Autodesk Fusion 360 part; units mm, degrees
(part 9 of 12)
  arc A1435 (77.1012, -97.0282) -> (78.6012, -97.0282) centre (77.8512, -97.0282) ccw
  arc A1436 (78.6012, -97.0282) -> (77.1012, -97.0282) centre (77.8512, -97.0282) ccw
  arc A1437 (77.1012, -97.0282) -> (78.6012, -97.0282) centre (77.8512, -97.0282) ccw
  arc A1438 (45.5811, -89.4082) -> (44.0811, -89.4082) centre (44.8311, -89.4082) ccw
  arc A1439 (44.0811, -89.4082) -> (45.5811, -89.4082) centre (44.8311, -89.4082) ccw
  arc A1440 (45.5811, -89.4082) -> (44.0811, -89.4082) centre (44.8311, -89.4082) ccw
  arc A1441 (44.0811, -89.4082) -> (45.5811, -89.4082) centre (44.8311, -89.4082) ccw
  arc A1442 (44.0811, -89.4082) -> (45.5811, -89.4082) centre (44.8311, -89.4082) ccw
  arc A1443 (45.5811, -89.4082) -> (44.0811, -89.4082) centre (44.8311, -89.4082) ccw
  arc A1444 (46.6211, -89.4082) -> (48.1211, -89.4082) centre (47.3711, -89.4082) ccw
  arc A1445 (48.1211, -89.4082) -> (46.6211, -89.4082) centre (47.3711, -89.4082) ccw
  arc A1446 (48.1211, -89.4082) -> (46.6211, -89.4082) centre (47.3711, -89.4082) ccw
  arc A1447 (46.6211, -89.4082) -> (48.1211, -89.4082) centre (47.3711, -89.4082) ccw
  arc A1448 (46.6211, -89.4082) -> (48.1211, -89.4082) centre (47.3711, -89.4082) ccw
  arc A1449 (48.1211, -89.4082) -> (46.6211, -89.4082) centre (47.3711, -89.4082) ccw
  arc A1450 (49.1611, -89.4082) -> (50.6611, -89.4082) centre (49.9111, -89.4082) ccw
  arc A1451 (50.6611, -89.4082) -> (49.1611, -89.4082) centre (49.9111, -89.4082) ccw
  arc A1452 (50.6611, -89.4082) -> (49.1611, -89.4082) centre (49.9111, -89.4082) ccw
  arc A1453 (49.1611, -89.4082) -> (50.6611, -89.4082) centre (49.9111, -89.4082) ccw
  arc A1454 (49.1611, -89.4082) -> (50.6611, -89.4082) centre (49.9111, -89.4082) ccw
  arc A1455 (50.6611, -89.4082) -> (49.1611, -89.4082) centre (49.9111, -89.4082) ccw
  arc A1456 (53.2011, -89.4082) -> (51.7011, -89.4082) centre (52.4511, -89.4082) ccw
  arc A1457 (51.7011, -89.4082) -> (53.2011, -89.4082) centre (52.4511, -89.4082) ccw
  arc A1458 (51.7011, -89.4082) -> (53.2011, -89.4082) centre (52.4511, -89.4082) ccw
  arc A1459 (53.2011, -89.4082) -> (51.7011, -89.4082) centre (52.4511, -89.4082) ccw
  arc A1460 (53.2011, -89.4082) -> (51.7011, -89.4082) centre (52.4511, -89.4082) ccw
  arc A1461 (51.7011, -89.4082) -> (53.2011, -89.4082) centre (52.4511, -89.4082) ccw
  arc A1462 (55.7411, -89.4082) -> (54.2411, -89.4082) centre (54.9911, -89.4082) ccw
  arc A1463 (54.2411, -89.4082) -> (55.7411, -89.4082) centre (54.9911, -89.4082) ccw
  arc A1464 (55.7411, -89.4082) -> (54.2411, -89.4082) centre (54.9911, -89.4082) ccw
  arc A1465 (54.2411, -89.4082) -> (55.7411, -89.4082) centre (54.9911, -89.4082) ccw
  arc A1466 (55.7411, -89.4082) -> (54.2411, -89.4082) centre (54.9911, -89.4082) ccw
  arc A1467 (54.2411, -89.4082) -> (55.7411, -89.4082) centre (54.9911, -89.4082) ccw
  arc A1468 (56.7811, -89.4082) -> (58.2811, -89.4082) centre (57.5311, -89.4082) ccw
  arc A1469 (58.2811, -89.4082) -> (56.7811, -89.4082) centre (57.5311, -89.4082) ccw
  arc A1470 (56.7811, -89.4082) -> (58.2811, -89.4082) centre (57.5311, -89.4082) ccw
  arc A1471 (58.2811, -89.4082) -> (56.7811, -89.4082) centre (57.5311, -89.4082) ccw
  arc A1472 (58.2811, -89.4082) -> (56.7811, -89.4082) centre (57.5311, -89.4082) ccw
  arc A1473 (56.7811, -89.4082) -> (58.2811, -89.4082) centre (57.5311, -89.4082) ccw
  arc A1474 (60.8211, -89.4082) -> (59.3211, -89.4082) centre (60.0711, -89.4082) ccw
  arc A1475 (59.3211, -89.4082) -> (60.8211, -89.4082) centre (60.0711, -89.4082) ccw
  arc A1476 (60.8211, -89.4082) -> (59.3211, -89.4082) centre (60.0711, -89.4082) ccw
  arc A1477 (59.3211, -89.4082) -> (60.8211, -89.4082) centre (60.0711, -89.4082) ccw
  arc A1478 (60.8211, -89.4082) -> (59.3211, -89.4082) centre (60.0711, -89.4082) ccw
  arc A1479 (59.3211, -89.4082) -> (60.8211, -89.4082) centre (60.0711, -89.4082) ccw
  arc A1480 (61.8611, -89.4082) -> (63.3611, -89.4082) centre (62.6111, -89.4082) ccw
  arc A1481 (63.3611, -89.4082) -> (61.8611, -89.4082) centre (62.6111, -89.4082) ccw
  arc A1482 (63.3611, -89.4082) -> (61.8611, -89.4082) centre (62.6111, -89.4082) ccw
  arc A1483 (61.8611, -89.4082) -> (63.3611, -89.4082) centre (62.6111, -89.4082) ccw
  arc A1484 (63.3611, -89.4082) -> (61.8611, -89.4082) centre (62.6111, -89.4082) ccw
  arc A1485 (61.8611, -89.4082) -> (63.3611, -89.4082) centre (62.6111, -89.4082) ccw
  arc A1486 (65.9011, -89.4082) -> (64.4011, -89.4082) centre (65.1511, -89.4082) ccw
  arc A1487 (64.4011, -89.4082) -> (65.9011, -89.4082) centre (65.1511, -89.4082) ccw
  arc A1488 (64.4011, -89.4082) -> (65.9011, -89.4082) centre (65.1511, -89.4082) ccw
  arc A1489 (65.9011, -89.4082) -> (64.4011, -89.4082) centre (65.1511, -89.4082) ccw
  arc A1490 (64.4011, -89.4082) -> (65.9011, -89.4082) centre (65.1511, -89.4082) ccw
  arc A1491 (65.9011, -89.4082) -> (64.4011, -89.4082) centre (65.1511, -89.4082) ccw
  arc A1492 (68.4411, -89.4082) -> (66.9411, -89.4082) centre (67.6911, -89.4082) ccw
  arc A1493 (66.9411, -89.4082) -> (68.4411, -89.4082) centre (67.6911, -89.4082) ccw
  arc A1494 (68.4411, -89.4082) -> (66.9411, -89.4082) centre (67.6911, -89.4082) ccw
  arc A1495 (66.9411, -89.4082) -> (68.4411, -89.4082) centre (67.6911, -89.4082) ccw
  arc A1496 (66.9411, -89.4082) -> (68.4411, -89.4082) centre (67.6911, -89.4082) ccw
  arc A1497 (68.4411, -89.4082) -> (66.9411, -89.4082) centre (67.6911, -89.4082) ccw
  arc A1498 (69.4811, -89.4082) -> (70.9811, -89.4082) centre (70.2311, -89.4082) ccw
  arc A1499 (70.9811, -89.4082) -> (69.4811, -89.4082) centre (70.2311, -89.4082) ccw
  arc A1500 (69.4811, -89.4082) -> (70.9811, -89.4082) centre (70.2311, -89.4082) ccw
  arc A1501 (70.9811, -89.4082) -> (69.4811, -89.4082) centre (70.2311, -89.4082) ccw
  arc A1502 (69.4811, -89.4082) -> (70.9811, -89.4082) centre (70.2311, -89.4082) ccw
  arc A1503 (70.9811, -89.4082) -> (69.4811, -89.4082) centre (70.2311, -89.4082) ccw
  arc A1504 (72.0211, -89.4082) -> (73.5211, -89.4082) centre (72.7711, -89.4082) ccw
  arc A1505 (73.5211, -89.4082) -> (72.0211, -89.4082) centre (72.7711, -89.4082) ccw
  arc A1506 (73.5211, -89.4082) -> (72.0211, -89.4082) centre (72.7711, -89.4082) ccw
  arc A1507 (72.0211, -89.4082) -> (73.5211, -89.4082) centre (72.7711, -89.4082) ccw
  arc A1508 (72.0211, -89.4082) -> (73.5211, -89.4082) centre (72.7711, -89.4082) ccw
  arc A1509 (73.5211, -89.4082) -> (72.0211, -89.4082) centre (72.7711, -89.4082) ccw
  arc A1510 (76.0612, -89.4082) -> (74.5612, -89.4082) centre (75.3112, -89.4082) ccw
  arc A1511 (74.5612, -89.4082) -> (76.0612, -89.4082) centre (75.3112, -89.4082) ccw
  arc A1512 (74.5612, -89.4082) -> (76.0612, -89.4082) centre (75.3112, -89.4082) ccw
  arc A1513 (76.0612, -89.4082) -> (74.5612, -89.4082) centre (75.3112, -89.4082) ccw
  arc A1514 (76.0612, -89.4082) -> (74.5612, -89.4082) centre (75.3112, -89.4082) ccw
  arc A1515 (74.5612, -89.4082) -> (76.0612, -89.4082) centre (75.3112, -89.4082) ccw
  line L256 (77.1012, -90.1582) -> (77.1012, -88.6582)
  line L257 (77.1012, -88.6582) -> (78.6012, -88.6582)
  line L258 (78.6012, -88.6582) -> (78.6012, -90.1582)
  line L259 (78.6012, -90.1582) -> (77.1012, -90.1582)
  line L260 (77.1012, -90.1582) -> (77.1012, -88.6582)
  line L261 (78.6012, -90.1582) -> (77.1012, -90.1582)
  line L262 (77.1012, -88.6582) -> (78.6012, -88.6582)
  line L263 (78.6012, -88.6582) -> (78.6012, -90.1582)
  line L264 (77.1012, -88.6582) -> (78.6012, -88.6582)
  line L265 (77.1012, -90.1582) -> (77.1012, -88.6582)
  line L266 (78.6012, -90.1582) -> (77.1012, -90.1582)
  line L267 (78.6012, -88.6582) -> (78.6012, -90.1582)
  arc A1516 (-155.9813, -117.1772) -> (-153.4413, -117.1772) centre (-154.7113, -117.1772) ccw
  arc A1517 (-153.4413, -117.1772) -> (-155.9813, -117.1772) centre (-154.7113, -117.1772) ccw
  arc A1518 (-153.4413, -117.1772) -> (-155.9813, -117.1772) centre (-154.7113, -117.1772) ccw
  arc A1519 (-155.9813, -117.1772) -> (-153.4413, -117.1772) centre (-154.7113, -117.1772) ccw
  arc A1520 (-153.4413, -117.1772) -> (-155.9813, -117.1772) centre (-154.7113, -117.1772) ccw
  arc A1521 (-155.9813, -117.1772) -> (-153.4413, -117.1772) centre (-154.7113, -117.1772) ccw
  arc A1522 (-159.7913, -119.7172) -> (-162.3313, -119.7172) centre (-161.0613, -119.7172) ccw
  arc A1523 (-162.3313, -119.7172) -> (-159.7913, -119.7172) centre (-161.0613, -119.7172) ccw
  arc A1524 (-159.7913, -119.7172) -> (-162.3313, -119.7172) centre (-161.0613, -119.7172) ccw
  arc A1525 (-162.3313, -119.7172) -> (-159.7913, -119.7172) centre (-161.0613, -119.7172) ccw
  arc A1526 (-159.7913, -119.7172) -> (-162.3313, -119.7172) centre (-161.0613, -119.7172) ccw
  arc A1527 (-162.3313, -119.7172) -> (-159.7913, -119.7172) centre (-161.0613, -119.7172) ccw
  arc A1528 (-110.7819, -117.1772) -> (-113.3219, -117.1772) centre (-112.0519, -117.1772) ccw
  arc A1529 (-113.3219, -117.1772) -> (-110.7819, -117.1772) centre (-112.0519, -117.1772) ccw
  arc A1530 (-113.3219, -117.1772) -> (-110.7819, -117.1772) centre (-112.0519, -117.1772) ccw
  arc A1531 (-110.7819, -117.1772) -> (-113.3219, -117.1772) centre (-112.0519, -117.1772) ccw
  arc A1532 (-113.3219, -117.1772) -> (-110.7819, -117.1772) centre (-112.0519, -117.1772) ccw
  arc A1533 (-110.7819, -117.1772) -> (-113.3219, -117.1772) centre (-112.0519, -117.1772) ccw
  arc A1534 (-117.132, -119.7172) -> (-119.672, -119.7172) centre (-118.402, -119.7172) ccw
  arc A1535 (-119.672, -119.7172) -> (-117.132, -119.7172) centre (-118.402, -119.7172) ccw
  arc A1536 (-117.132, -119.7172) -> (-119.672, -119.7172) centre (-118.402, -119.7172) ccw
  arc A1537 (-119.672, -119.7172) -> (-117.132, -119.7172) centre (-118.402, -119.7172) ccw
  arc A1538 (-117.132, -119.7172) -> (-119.672, -119.7172) centre (-118.402, -119.7172) ccw
  arc A1539 (-119.672, -119.7172) -> (-117.132, -119.7172) centre (-118.402, -119.7172) ccw
  arc A1540 (-80.7819, -117.1772) -> (-83.3219, -117.1772) centre (-82.0519, -117.1772) ccw
  arc A1541 (-83.3219, -117.1772) -> (-80.7819, -117.1772) centre (-82.0519, -117.1772) ccw
  arc A1542 (-83.3219, -117.1772) -> (-80.7819, -117.1772) centre (-82.0519, -117.1772) ccw
  arc A1543 (-80.7819, -117.1772) -> (-83.3219, -117.1772) centre (-82.0519, -117.1772) ccw
  arc A1544 (-83.3219, -117.1772) -> (-80.7819, -117.1772) centre (-82.0519, -117.1772) ccw
  arc A1545 (-80.7819, -117.1772) -> (-83.3219, -117.1772) centre (-82.0519, -117.1772) ccw
  arc A1546 (-89.672, -119.7172) -> (-87.132, -119.7172) centre (-88.402, -119.7172) ccw
  arc A1547 (-87.132, -119.7172) -> (-89.672, -119.7172) centre (-88.402, -119.7172) ccw
  arc A1548 (-87.132, -119.7172) -> (-89.672, -119.7172) centre (-88.402, -119.7172) ccw
  arc A1549 (-89.672, -119.7172) -> (-87.132, -119.7172) centre (-88.402, -119.7172) ccw
  arc A1550 (-87.132, -119.7172) -> (-89.672, -119.7172) centre (-88.402, -119.7172) ccw
  arc A1551 (-89.672, -119.7172) -> (-87.132, -119.7172) centre (-88.402, -119.7172) ccw
  arc A1552 (-53.3219, -117.1772) -> (-50.7819, -117.1772) centre (-52.0519, -117.1772) ccw
  arc A1553 (-50.7819, -117.1772) -> (-53.3219, -117.1772) centre (-52.0519, -117.1772) ccw
  arc A1554 (-50.7819, -117.1772) -> (-53.3219, -117.1772) centre (-52.0519, -117.1772) ccw
  arc A1555 (-53.3219, -117.1772) -> (-50.7819, -117.1772) centre (-52.0519, -117.1772) ccw
  arc A1556 (-50.7819, -117.1772) -> (-53.3219, -117.1772) centre (-52.0519, -117.1772) ccw
  arc A1557 (-53.3219, -117.1772) -> (-50.7819, -117.1772) centre (-52.0519, -117.1772) ccw
  arc A1558 (-57.132, -119.7172) -> (-59.672, -119.7172) centre (-58.402, -119.7172) ccw
  arc A1559 (-59.672, -119.7172) -> (-57.132, -119.7172) centre (-58.402, -119.7172) ccw
  arc A1560 (-57.132, -119.7172) -> (-59.672, -119.7172) centre (-58.402, -119.7172) ccw
  arc A1561 (-59.672, -119.7172) -> (-57.132, -119.7172) centre (-58.402, -119.7172) ccw
  arc A1562 (-57.132, -119.7172) -> (-59.672, -119.7172) centre (-58.402, -119.7172) ccw
  arc A1563 (-59.672, -119.7172) -> (-57.132, -119.7172) centre (-58.402, -119.7172) ccw
  arc A1564 (-23.3219, -117.1772) -> (-20.7819, -117.1772) centre (-22.0519, -117.1772) ccw
  arc A1565 (-20.7819, -117.1772) -> (-23.3219, -117.1772) centre (-22.0519, -117.1772) ccw
  arc A1566 (-20.7819, -117.1772) -> (-23.3219, -117.1772) centre (-22.0519, -117.1772) ccw
  arc A1567 (-23.3219, -117.1772) -> (-20.7819, -117.1772) centre (-22.0519, -117.1772) ccw
  arc A1568 (-20.7819, -117.1772) -> (-23.3219, -117.1772) centre (-22.0519, -117.1772) ccw
  arc A1569 (-23.3219, -117.1772) -> (-20.7819, -117.1772) centre (-22.0519, -117.1772) ccw
  arc A1570 (-27.132, -119.7172) -> (-29.672, -119.7172) centre (-28.402, -119.7172) ccw
  arc A1571 (-29.672, -119.7172) -> (-27.132, -119.7172) centre (-28.402, -119.7172) ccw
  arc A1572 (-27.132, -119.7172) -> (-29.672, -119.7172) centre (-28.402, -119.7172) ccw
  arc A1573 (-29.672, -119.7172) -> (-27.132, -119.7172) centre (-28.402, -119.7172) ccw
  arc A1574 (-27.132, -119.7172) -> (-29.672, -119.7172) centre (-28.402, -119.7172) ccw
  arc A1575 (-29.672, -119.7172) -> (-27.132, -119.7172) centre (-28.402, -119.7172) ccw
  arc A1576 (6.6781, -117.1772) -> (9.2181, -117.1772) centre (7.9481, -117.1772) ccw
  arc A1577 (9.2181, -117.1772) -> (6.6781, -117.1772) centre (7.9481, -117.1772) ccw
  arc A1578 (6.6781, -117.1772) -> (9.2181, -117.1772) centre (7.9481, -117.1772) ccw
  arc A1579 (9.2181, -117.1772) -> (6.6781, -117.1772) centre (7.9481, -117.1772) ccw
  arc A1580 (6.6781, -117.1772) -> (9.2181, -117.1772) centre (7.9481, -117.1772) ccw
  arc A1581 (9.2181, -117.1772) -> (6.6781, -117.1772) centre (7.9481, -117.1772) ccw
  arc A1582 (2.868, -119.7172) -> (0.328, -119.7172) centre (1.598, -119.7172) ccw
  arc A1583 (0.328, -119.7172) -> (2.868, -119.7172) centre (1.598, -119.7172) ccw
  arc A1584 (2.868, -119.7172) -> (0.328, -119.7172) centre (1.598, -119.7172) ccw
  arc A1585 (0.328, -119.7172) -> (2.868, -119.7172) centre (1.598, -119.7172) ccw
  arc A1586 (2.868, -119.7172) -> (0.328, -119.7172) centre (1.598, -119.7172) ccw
  arc A1587 (0.328, -119.7172) -> (2.868, -119.7172) centre (1.598, -119.7172) ccw
  arc A1588 (36.6781, -117.1772) -> (39.2181, -117.1772) centre (37.9481, -117.1772) ccw
  arc A1589 (39.2181, -117.1772) -> (36.6781, -117.1772) centre (37.9481, -117.1772) ccw
  arc A1590 (39.2181, -117.1772) -> (36.6781, -117.1772) centre (37.9481, -117.1772) ccw
  arc A1591 (36.6781, -117.1772) -> (39.2181, -117.1772) centre (37.9481, -117.1772) ccw
  arc A1592 (36.6781, -117.1772) -> (39.2181, -117.1772) centre (37.9481, -117.1772) ccw
  arc A1593 (39.2181, -117.1772) -> (36.6781, -117.1772) centre (37.9481, -117.1772) ccw
  arc A1594 (32.868, -119.7172) -> (30.328, -119.7172) centre (31.598, -119.7172) ccw
  arc A1595 (30.328, -119.7172) -> (32.868, -119.7172) centre (31.598, -119.7172) ccw
  arc A1596 (30.328, -119.7172) -> (32.868, -119.7172) centre (31.598, -119.7172) ccw
  arc A1597 (32.868, -119.7172) -> (30.328, -119.7172) centre (31.598, -119.7172) ccw
  arc A1598 (30.328, -119.7172) -> (32.868, -119.7172) centre (31.598, -119.7172) ccw
  arc A1599 (32.868, -119.7172) -> (30.328, -119.7172) centre (31.598, -119.7172) ccw
  line L268 (-165.2393, 23.796) -> (-166.7393, 23.796)
  line L269 (-166.7393, 23.796) -> (-166.7393, 26.296)
  line L270 (-166.7393, 26.296) -> (-165.2393, 26.296)
  line L271 (-165.2393, 26.296) -> (-165.2393, 23.796)
  line L272 (-166.7393, 26.296) -> (-165.2393, 26.296)
  line L273 (-165.2393, 26.296) -> (-165.2393, 23.796)
  line L274 (-166.7393, 23.796) -> (-166.7393, 26.296)
  line L275 (-165.2393, 23.796) -> (-166.7393, 23.796)
  line L276 (-166.7393, 26.296) -> (-165.2393, 26.296)
  line L277 (-166.7393, 23.796) -> (-166.7393, 26.296)
  line L278 (-165.2393, 26.296) -> (-165.2393, 23.796)
  line L279 (-165.2393, 23.796) -> (-166.7393, 23.796)
  line L280 (-169.6488, 22.7962) -> (-171.1488, 22.7962)
  line L281 (-169.6488, 25.2962) -> (-169.6488, 22.7962)
  line L282 (-171.1488, 25.2962) -> (-169.6488, 25.2962)
  line L283 (-171.1488, 22.7962) -> (-171.1488, 25.2962)
  line L284 (-169.6488, 22.7962) -> (-171.1488, 22.7962)
  line L285 (-171.1488, 25.2962) -> (-169.6488, 25.2962)
  line L286 (-171.1488, 22.7962) -> (-171.1488, 25.2962)
  line L287 (-169.6488, 25.2962) -> (-169.6488, 22.7962)
  line L288 (-171.1488, 22.7962) -> (-171.1488, 25.2962)
  line L289 (-169.6488, 25.2962) -> (-169.6488, 22.7962)
  line L290 (-171.1488, 25.2962) -> (-169.6488, 25.2962)
  line L291 (-169.6488, 22.7962) -> (-171.1488, 22.7962)
  line L292 (-165.2393, 27.796) -> (-166.7393, 27.796)
  line L293 (-166.7393, 30.296) -> (-165.2393, 30.296)
  line L294 (-166.7393, 27.796) -> (-166.7393, 30.296)
  line L295 (-165.2393, 30.296) -> (-165.2393, 27.796)
  line L296 (-166.7393, 27.796) -> (-166.7393, 30.296)
  line L297 (-165.2393, 30.296) -> (-165.2393, 27.796)
  line L298 (-166.7393, 30.296) -> (-165.2393, 30.296)
  line L299 (-165.2393, 27.796) -> (-166.7393, 27.796)
  line L300 (-165.2393, 27.796) -> (-166.7393, 27.796)
  line L301 (-165.2393, 30.296) -> (-165.2393, 27.796)
  line L302 (-166.7393, 27.796) -> (-166.7393, 30.296)
  line L303 (-166.7393, 30.296) -> (-165.2393, 30.296)
  line L304 (-165.2393, 31.1351) -> (-166.7393, 31.1351)
  line L305 (-166.7393, 33.6351) -> (-165.2393, 33.6351)
  line L306 (-165.2393, 33.6351) -> (-165.2393, 31.1351)
  line L307 (-166.7393, 31.1351) -> (-166.7393, 33.6351)
  line L308 (-166.7393, 33.6351) -> (-165.2393, 33.6351)
  line L309 (-166.7393, 31.1351) -> (-166.7393, 33.6351)
  line L310 (-165.2393, 33.6351) -> (-165.2393, 31.1351)
  line L311 (-165.2393, 31.1351) -> (-166.7393, 31.1351)
  line L312 (-165.2393, 31.1351) -> (-166.7393, 31.1351)
  line L313 (-166.7393, 31.1351) -> (-166.7393, 33.6351)
  line L314 (-166.7393, 33.6351) -> (-165.2393, 33.6351)
  line L315 (-165.2393, 33.6351) -> (-165.2393, 31.1351)
  arc A1600 (79.5553, -109.509) -> (80.1653, -109.509) centre (79.8603, -109.509) ccw
  arc A1601 (80.1653, -109.509) -> (79.5553, -109.509) centre (79.8603, -109.509) ccw
  arc A1602 (81.2321, -118.3868) -> (80.6221, -118.3868) centre (80.9271, -118.3868) ccw
  arc A1603 (80.6221, -118.3868) -> (81.2321, -118.3868) centre (80.9271, -118.3868) ccw
  arc A1604 (-137.7096, -37.6617) -> (-137.0996, -37.6617) centre (-137.4046, -37.6617) ccw
  arc A1605 (-137.0996, -37.6617) -> (-137.7096, -37.6617) centre (-137.4046, -37.6617) ccw
  arc A1606 (31.9479, -125.0968) -> (31.3379, -125.0968) centre (31.6429, -125.0968) ccw
  arc A1607 (31.3379, -125.0968) -> (31.9479, -125.0968) centre (31.6429, -125.0968) ccw
  arc A1608 (-96.655, -5.6767) -> (-96.045, -5.6767) centre (-96.35, -5.6767) ccw
  arc A1609 (-96.045, -5.6767) -> (-96.655, -5.6767) centre (-96.35, -5.6767) ccw
  arc A1610 (-131.4781, -63.5725) -> (-132.0881, -63.5725) centre (-131.7831, -63.5725) ccw
  arc A1611 (-132.0881, -63.5725) -> (-131.4781, -63.5725) centre (-131.7831, -63.5725) ccw
  arc A1612 (-72.0881, -63.5296) -> (-71.4781, -63.5296) centre (-71.7831, -63.5296) ccw
  arc A1613 (-71.4781, -63.5296) -> (-72.0881, -63.5296) centre (-71.7831, -63.5296) ccw
  arc A1614 (0.838, -62.3231) -> (1.448, -62.3231) centre (1.143, -62.3231) ccw
  arc A1615 (1.448, -62.3231) -> (0.838, -62.3231) centre (1.143, -62.3231) ccw
  arc A1616 (39.8499, -119.5512) -> (40.4599, -119.5512) centre (40.1549, -119.5512) ccw
  arc A1617 (40.4599, -119.5512) -> (39.8499, -119.5512) centre (40.1549, -119.5512) ccw
  arc A1618 (1.9408, -125.0963) -> (1.3308, -125.0963) centre (1.6358, -125.0963) ccw
  arc A1619 (1.3308, -125.0963) -> (1.9408, -125.0963) centre (1.6358, -125.0963) ccw
  arc A1620 (80.7008, -116.9472) -> (81.3108, -116.9472) centre (81.0058, -116.9472) ccw
  arc A1621 (81.3108, -116.9472) -> (80.7008, -116.9472) centre (81.0058, -116.9472) ccw
  arc A1622 (81.4247, 15.3665) -> (82.0347, 15.3665) centre (81.7297, 15.3665) ccw
  arc A1623 (82.0347, 15.3665) -> (81.4247, 15.3665) centre (81.7297, 15.3665) ccw
  arc A1624 (78.6972, -115.5227) -> (78.0872, -115.5227) centre (78.3922, -115.5227) ccw
  arc A1625 (78.0872, -115.5227) -> (78.6972, -115.5227) centre (78.3922, -115.5227) ccw
  arc A1626 (77.2464, -117.8524) -> (77.8564, -117.8524) centre (77.5514, -117.8524) ccw
  arc A1627 (77.8564, -117.8524) -> (77.2464, -117.8524) centre (77.5514, -117.8524) ccw
  arc A1628 (75.8926, -85.9792) -> (76.5026, -85.9792) centre (76.1976, -85.9792) ccw
  arc A1629 (76.5026, -85.9792) -> (75.8926, -85.9792) centre (76.1976, -85.9792) ccw
  arc A1630 (78.5926, -85.9792) -> (79.2026, -85.9792) centre (78.8976, -85.9792) ccw
  arc A1631 (79.2026, -85.9792) -> (78.5926, -85.9792) centre (78.8976, -85.9792) ccw
  arc A1632 (77.8361, -112.2817) -> (77.2261, -112.2817) centre (77.5311, -112.2817) ccw
  arc A1633 (77.2261, -112.2817) -> (77.8361, -112.2817) centre (77.5311, -112.2817) ccw
  arc A1634 (73.6218, -112.2817) -> (74.2319, -112.2817) centre (73.9268, -112.2817) ccw
  arc A1635 (74.2319, -112.2817) -> (73.6218, -112.2817) centre (73.9268, -112.2817) ccw
  arc A1636 (74.2319, -116.9995) -> (73.6218, -116.9995) centre (73.9268, -116.9995) ccw
  arc A1637 (73.6218, -116.9995) -> (74.2319, -116.9995) centre (73.9268, -116.9995) ccw
  arc A1638 (45.1945, -78.1687) -> (44.5845, -78.1687) centre (44.8895, -78.1687) ccw
  arc A1639 (44.5845, -78.1687) -> (45.1945, -78.1687) centre (44.8895, -78.1687) ccw
  arc A1640 (63.0482, -60.3089) -> (62.4382, -60.3089) centre (62.7432, -60.3089) ccw
  arc A1641 (62.4382, -60.3089) -> (63.0482, -60.3089) centre (62.7432, -60.3089) ccw
  arc A1642 (57.8764, -64.1397) -> (58.4864, -64.1397) centre (58.1814, -64.1397) ccw
  arc A1643 (58.4864, -64.1397) -> (57.8764, -64.1397) centre (58.1814, -64.1397) ccw
  arc A1644 (25.8923, -33.4412) -> (25.2822, -33.4412) centre (25.5872, -33.4412) ccw
  arc A1645 (25.2822, -33.4412) -> (25.8923, -33.4412) centre (25.5872, -33.4412) ccw
  arc A1646 (54.8846, -5.5405) -> (54.2746, -5.5405) centre (54.5796, -5.5405) ccw
  arc A1647 (54.2746, -5.5405) -> (54.8846, -5.5405) centre (54.5796, -5.5405) ccw
  arc A1648 (43.4745, 19.9916) -> (44.0845, 19.9916) centre (43.7795, 19.9916) ccw
  arc A1649 (44.0845, 19.9916) -> (43.4745, 19.9916) centre (43.7795, 19.9916) ccw
  arc A1650 (29.6902, 19.9916) -> (30.3002, 19.9916) centre (29.9952, 19.9916) ccw
  arc A1651 (30.3002, 19.9916) -> (29.6902, 19.9916) centre (29.9952, 19.9916) ccw
  arc A1652 (54.5007, -6.8923) -> (55.1107, -6.8923) centre (54.8057, -6.8923) ccw
  arc A1653 (55.1107, -6.8923) -> (54.5007, -6.8923) centre (54.8057, -6.8923) ccw
  arc A1654 (18.772, -34.9096) -> (19.382, -34.9096) centre (19.077, -34.9096) ccw
  arc A1655 (19.382, -34.9096) -> (18.772, -34.9096) centre (19.077, -34.9096) ccw
  arc A1656 (48.8314, -36.415) -> (49.4414, -36.415) centre (49.1364, -36.415) ccw
  arc A1657 (49.4414, -36.415) -> (48.8314, -36.415) centre (49.1364, -36.415) ccw
  arc A1658 (-161.534, -49.4031) -> (-162.144, -49.4031) centre (-161.839, -49.4031) ccw
  arc A1659 (-162.144, -49.4031) -> (-161.534, -49.4031) centre (-161.839, -49.4031) ccw
  arc A1660 (-178.0948, -46.4056) -> (-178.7048, -46.4056) centre (-178.3998, -46.4056) ccw
  arc A1661 (-178.7048, -46.4056) -> (-178.0948, -46.4056) centre (-178.3998, -46.4056) ccw
  arc A1662 (80.3101, -110.2962) -> (79.7001, -110.2962) centre (80.0051, -110.2962) ccw
  arc A1663 (79.7001, -110.2962) -> (80.3101, -110.2962) centre (80.0051, -110.2962) ccw
  arc A1664 (51.4324, -115.889) -> (52.0424, -115.889) centre (51.7374, -115.889) ccw
  arc A1665 (52.0424, -115.889) -> (51.4324, -115.889) centre (51.7374, -115.889) ccw
  arc A1666 (81.4124, -115.2316) -> (80.8024, -115.2316) centre (81.1074, -115.2316) ccw
  arc A1667 (80.8024, -115.2316) -> (81.4124, -115.2316) centre (81.1074, -115.2316) ccw
  arc A1668 (-184.8118, 17.1631) -> (-185.4218, 17.1631) centre (-185.1168, 17.1631) ccw
  arc A1669 (-185.4218, 17.1631) -> (-184.8118, 17.1631) centre (-185.1168, 17.1631) ccw
  arc A1670 (-168.57, 17.1631) -> (-169.18, 17.1631) centre (-168.875, 17.1631) ccw
  arc A1671 (-169.18, 17.1631) -> (-168.57, 17.1631) centre (-168.875, 17.1631) ccw
  arc A1672 (45.5374, 16.3147) -> (44.9274, 16.3147) centre (45.2324, 16.3147) ccw
  arc A1673 (44.9274, 16.3147) -> (45.5374, 16.3147) centre (45.2324, 16.3147) ccw
  arc A1674 (68.2933, -38.6081) -> (67.6833, -38.6081) centre (67.9883, -38.6081) ccw
  arc A1675 (67.6833, -38.6081) -> (68.2933, -38.6081) centre (67.9883, -38.6081) ccw
  arc A1676 (-155.7475, 20.8895) -> (-155.1375, 20.8895) centre (-155.4425, 20.8895) ccw
  arc A1677 (-155.1375, 20.8895) -> (-155.7475, 20.8895) centre (-155.4425, 20.8895) ccw
  arc A1678 (-124.2998, 23.0592) -> (-124.9098, 23.0592) centre (-124.6048, 23.0592) ccw
  arc A1679 (-124.9098, 23.0592) -> (-124.2998, 23.0592) centre (-124.6048, 23.0592) ccw
  arc A1680 (-122.3903, -27.0211) -> (-121.7803, -27.0211) centre (-122.0853, -27.0211) ccw
  arc A1681 (-121.7803, -27.0211) -> (-122.3903, -27.0211) centre (-122.0853, -27.0211) ccw
  arc A1682 (72.9542, -37.3381) -> (72.3442, -37.3381) centre (72.6492, -37.3381) ccw
  arc A1683 (72.3442, -37.3381) -> (72.9542, -37.3381) centre (72.6492, -37.3381) ccw
  arc A1684 (-91.3126, -43.2421) -> (-90.7026, -43.2421) centre (-91.0076, -43.2421) ccw
  arc A1685 (-90.7026, -43.2421) -> (-91.3126, -43.2421) centre (-91.0076, -43.2421) ccw
  arc A1686 (-88.2633, -46.4056) -> (-87.6533, -46.4056) centre (-87.9583, -46.4056) ccw
  arc A1687 (-87.6533, -46.4056) -> (-88.2633, -46.4056) centre (-87.9583, -46.4056) ccw
  arc A1688 (-68.0165, 28.6035) -> (-67.4065, 28.6035) centre (-67.7115, 28.6035) ccw
  arc A1689 (-67.4065, 28.6035) -> (-68.0165, 28.6035) centre (-67.7115, 28.6035) ccw
  arc A1690 (-39.0957, 27.985) -> (-38.4857, 27.985) centre (-38.7907, 27.985) ccw
  arc A1691 (-38.4857, 27.985) -> (-39.0957, 27.985) centre (-38.7907, 27.985) ccw
  arc A1692 (36.3576, -47.3741) -> (35.7476, -47.3741) centre (36.0526, -47.3741) ccw
  arc A1693 (35.7476, -47.3741) -> (36.3576, -47.3741) centre (36.0526, -47.3741) ccw
  arc A1694 (-37.3323, 28.636) -> (-37.9423, 28.636) centre (-37.6373, 28.636) ccw
  arc A1695 (-37.9423, 28.636) -> (-37.3323, 28.636) centre (-37.6373, 28.636) ccw
  arc A1696 (-17.5237, 28.0457) -> (-16.9137, 28.0457) centre (-17.2187, 28.0457) ccw
  arc A1697 (-16.9137, 28.0457) -> (-17.5237, 28.0457) centre (-17.2187, 28.0457) ccw
  arc A1698 (42.9314, -51.3081) -> (42.3214, -51.3081) centre (42.6264, -51.3081) ccw
  arc A1699 (42.3214, -51.3081) -> (42.9314, -51.3081) centre (42.6264, -51.3081) ccw
  arc A1700 (50.0561, -50.0381) -> (49.4461, -50.0381) centre (49.7511, -50.0381) ccw
  arc A1701 (49.4461, -50.0381) -> (50.0561, -50.0381) centre (49.7511, -50.0381) ccw
  arc A1702 (20.6511, 22.5339) -> (21.2611, 22.5339) centre (20.9561, 22.5339) ccw
  arc A1703 (21.2611, 22.5339) -> (20.6511, 22.5339) centre (20.9561, 22.5339) ccw
  arc A1704 (-115.2868, 22.5339) -> (-115.8968, 22.5339) centre (-115.5918, 22.5339) ccw
  arc A1705 (-115.8968, 22.5339) -> (-115.2868, 22.5339) centre (-115.5918, 22.5339) ccw
  arc A1706 (-117.4115, 5.461) -> (-118.0215, 5.461) centre (-117.7165, 5.461) ccw
  arc A1707 (-118.0215, 5.461) -> (-117.4115, 5.461) centre (-117.7165, 5.461) ccw
  arc A1708 (-177.5561, 5.461) -> (-178.1661, 5.461) centre (-177.8611, 5.461) ccw
  arc A1709 (-178.1661, 5.461) -> (-177.5561, 5.461) centre (-177.8611, 5.461) ccw
  arc A1710 (67.6732, -73.8407) -> (68.2832, -73.8407) centre (67.9782, -73.8407) ccw
  arc A1711 (68.2832, -73.8407) -> (67.6732, -73.8407) centre (67.9782, -73.8407) ccw
  arc A1712 (76.3447, -73.8407) -> (76.9547, -73.8407) centre (76.6497, -73.8407) ccw
  arc A1713 (76.9547, -73.8407) -> (76.3447, -73.8407) centre (76.6497, -73.8407) ccw
  arc A1714 (77.9987, -114.937) -> (77.3887, -114.937) centre (77.6937, -114.937) ccw
  arc A1715 (77.3887, -114.937) -> (77.9987, -114.937) centre (77.6937, -114.937) ccw
  arc A1716 (-116.0229, -5.8308) -> (-116.6329, -5.8308) centre (-116.3279, -5.8308) ccw
  arc A1717 (-116.6329, -5.8308) -> (-116.0229, -5.8308) centre (-116.3279, -5.8308) ccw
  arc A1718 (-90.3967, -94.2073) -> (-89.7867, -94.2073) centre (-90.0917, -94.2073) ccw
  arc A1719 (-89.7867, -94.2073) -> (-90.3967, -94.2073) centre (-90.0917, -94.2073) ccw
  arc A1720 (-155.1375, -9.1105) -> (-155.7475, -9.1105) centre (-155.4425, -9.1105) ccw
  arc A1721 (-155.7475, -9.1105) -> (-155.1375, -9.1105) centre (-155.4425, -9.1105) ccw
  arc A1722 (-124.6738, -6.8494) -> (-124.0638, -6.8494) centre (-124.3688, -6.8494) ccw
  arc A1723 (-124.0638, -6.8494) -> (-124.6738, -6.8494) centre (-124.3688, -6.8494) ccw
  arc A1724 (-148.5769, -6.4173) -> (-149.1869, -6.4173) centre (-148.8819, -6.4173) ccw
  arc A1725 (-149.1869, -6.4173) -> (-148.5769, -6.4173) centre (-148.8819, -6.4173) ccw
  arc A1726 (52.7688, -22.0432) -> (52.1588, -22.0432) centre (52.4638, -22.0432) ccw
  arc A1727 (52.1588, -22.0432) -> (52.7688, -22.0432) centre (52.4638, -22.0432) ccw
  arc A1728 (68.2066, -95.077) -> (68.8166, -95.077) centre (68.5116, -95.077) ccw
  arc A1729 (68.8166, -95.077) -> (68.2066, -95.077) centre (68.5116, -95.077) ccw
  arc A1730 (-126.3953, 2.5314) -> (-127.0053, 2.5314) centre (-126.7003, 2.5314) ccw
  arc A1731 (-127.0053, 2.5314) -> (-126.3953, 2.5314) centre (-126.7003, 2.5314) ccw
  arc A1732 (-96.0401, 2.5314) -> (-95.4301, 2.5314) centre (-95.7351, 2.5314) ccw
  arc A1733 (-95.4301, 2.5314) -> (-96.0401, 2.5314) centre (-95.7351, 2.5314) ccw
  arc A1734 (72.5758, -32.4915) -> (71.9658, -32.4915) centre (72.2708, -32.4915) ccw
  arc A1735 (71.9658, -32.4915) -> (72.5758, -32.4915) centre (72.2708, -32.4915) ccw
  arc A1736 (-64.3305, -13.1039) -> (-64.9405, -13.1039) centre (-64.6355, -13.1039) ccw
  arc A1737 (-64.9405, -13.1039) -> (-64.3305, -13.1039) centre (-64.6355, -13.1039) ccw
  arc A1738 (-30.0519, -7.1473) -> (-30.6619, -7.1473) centre (-30.3569, -7.1473) ccw
  arc A1739 (-30.6619, -7.1473) -> (-30.0519, -7.1473) centre (-30.3569, -7.1473) ccw
  arc A1740 (-50.7364, -97.062) -> (-51.3464, -97.062) centre (-51.0414, -97.062) ccw
  arc A1741 (-51.3464, -97.062) -> (-50.7364, -97.062) centre (-51.0414, -97.062) ccw
  arc A1742 (-28.9723, -17.8428) -> (-28.3623, -17.8428) centre (-28.6673, -17.8428) ccw
  arc A1743 (-28.3623, -17.8428) -> (-28.9723, -17.8428) centre (-28.6673, -17.8428) ccw
  arc A1744 (14.2044, -17.8428) -> (13.5944, -17.8428) centre (13.8994, -17.8428) ccw
  arc A1745 (13.5944, -17.8428) -> (14.2044, -17.8428) centre (13.8994, -17.8428) ccw
  arc A1746 (11.0779, -13.8291) -> (10.4679, -13.8291) centre (10.7729, -13.8291) ccw
  arc A1747 (10.4679, -13.8291) -> (11.0779, -13.8291) centre (10.7729, -13.8291) ccw
  arc A1748 (53.8255, -13.8291) -> (53.2154, -13.8291) centre (53.5204, -13.8291) ccw
  arc A1749 (53.2154, -13.8291) -> (53.8255, -13.8291) centre (53.5204, -13.8291) ccw
  arc A1750 (43.3069, -47.7371) -> (43.9169, -47.7371) centre (43.6119, -47.7371) ccw
  arc A1751 (43.9169, -47.7371) -> (43.3069, -47.7371) centre (43.6119, -47.7371) ccw
  arc A1752 (47.1829, -24.9017) -> (47.7929, -24.9017) centre (47.4879, -24.9017) ccw
  arc A1753 (47.7929, -24.9017) -> (47.1829, -24.9017) centre (47.4879, -24.9017) ccw
  arc A1754 (-185.1149, -24.9017) -> (-185.7249, -24.9017) centre (-185.4199, -24.9017) ccw
  arc A1755 (-185.7249, -24.9017) -> (-185.1149, -24.9017) centre (-185.4199, -24.9017) ccw
  arc A1756 (74.0795, -3.683) -> (73.4694, -3.683) centre (73.7744, -3.683) ccw
  arc A1757 (73.4694, -3.683) -> (74.0795, -3.683) centre (73.7744, -3.683) ccw
  arc A1758 (-197.0719, -41.0805) -> (-197.6819, -41.0805) centre (-197.3769, -41.0805) ccw
  arc A1759 (-197.6819, -41.0805) -> (-197.0719, -41.0805) centre (-197.3769, -41.0805) ccw
  arc A1760 (-186.0511, -41.0805) -> (-186.6611, -41.0805) centre (-186.3561, -41.0805) ccw
  arc A1761 (-186.6611, -41.0805) -> (-186.0511, -41.0805) centre (-186.3561, -41.0805) ccw
  arc A1762 (-167.6819, -41.0805) -> (-167.0719, -41.0805) centre (-167.3769, -41.0805) ccw
  arc A1763 (-167.0719, -41.0805) -> (-167.6819, -41.0805) centre (-167.3769, -41.0805) ccw
  arc A1764 (-155.5583, -41.0805) -> (-156.1684, -41.0805) centre (-155.8633, -41.0805) ccw
  arc A1765 (-156.1684, -41.0805) -> (-155.5583, -41.0805) centre (-155.8633, -41.0805) ccw
  arc A1766 (-136.6129, -42.1496) -> (-136.0028, -42.1496) centre (-136.3078, -42.1496) ccw
  arc A1767 (-136.0028, -42.1496) -> (-136.6129, -42.1496) centre (-136.3078, -42.1496) ccw
  arc A1768 (-100.4605, -42.1496) -> (-99.8504, -42.1496) centre (-100.1554, -42.1496) ccw
  arc A1769 (-99.8504, -42.1496) -> (-100.4605, -42.1496) centre (-100.1554, -42.1496) ccw
  arc A1770 (-106.7394, -40.8397) -> (-107.3495, -40.8397) centre (-107.0445, -40.8397) ccw
  arc A1771 (-107.3495, -40.8397) -> (-106.7394, -40.8397) centre (-107.0445, -40.8397) ccw
  arc A1772 (-70.5265, -40.4031) -> (-69.9165, -40.4031) centre (-70.2215, -40.4031) ccw
  arc A1773 (-69.9165, -40.4031) -> (-70.5265, -40.4031) centre (-70.2215, -40.4031) ccw
  arc A1774 (-79.1155, -40.9294) -> (-78.5055, -40.9294) centre (-78.8105, -40.9294) ccw
  arc A1775 (-78.5055, -40.9294) -> (-79.1155, -40.9294) centre (-78.8105, -40.9294) ccw
  arc A1776 (-41.4113, -38.5108) -> (-42.0213, -38.5108) centre (-41.7163, -38.5108) ccw
  arc A1777 (-42.0213, -38.5108) -> (-41.4113, -38.5108) centre (-41.7163, -38.5108) ccw
  arc A1778 (-20.8144, -30.2896) -> (-21.4244, -30.2896) centre (-21.1194, -30.2896) ccw
  arc A1779 (-21.4244, -30.2896) -> (-20.8144, -30.2896) centre (-21.1194, -30.2896) ccw
  arc A1780 (-18.439, -94.8771) -> (-19.049, -94.8771) centre (-18.744, -94.8771) ccw
  arc A1781 (-19.049, -94.8771) -> (-18.439, -94.8771) centre (-18.744, -94.8771) ccw
  arc A1782 (-41.8657, -40.8832) -> (-42.4757, -40.8832) centre (-42.1707, -40.8832) ccw
  arc A1783 (-42.4757, -40.8832) -> (-41.8657, -40.8832) centre (-42.1707, -40.8832) ccw
  arc A1784 (-11.6229, -38.3053) -> (-12.2329, -38.3053) centre (-11.9279, -38.3053) ccw
  arc A1785 (-12.2329, -38.3053) -> (-11.6229, -38.3053) centre (-11.9279, -38.3053) ccw
  arc A1786 (-48.9647, -27.7981) -> (-49.5748, -27.7981) centre (-49.2697, -27.7981) ccw
  arc A1787 (-49.5748, -27.7981) -> (-48.9647, -27.7981) centre (-49.2697, -27.7981) ccw
  arc A1788 (-42.336, -99.7239) -> (-41.726, -99.7239) centre (-42.031, -99.7239) ccw
  arc A1789 (-41.726, -99.7239) -> (-42.336, -99.7239) centre (-42.031, -99.7239) ccw
  arc A1790 (62.2401, -99.7239) -> (62.8501, -99.7239) centre (62.5451, -99.7239) ccw
  arc A1791 (62.8501, -99.7239) -> (62.2401, -99.7239) centre (62.5451, -99.7239) ccw
  arc A1792 (42.8501, -30.299) -> (42.2401, -30.299) centre (42.5451, -30.299) ccw
  arc A1793 (42.2401, -30.299) -> (42.8501, -30.299) centre (42.5451, -30.299) ccw
  arc A1794 (16.022, -42.1496) -> (15.412, -42.1496) centre (15.717, -42.1496) ccw
  arc A1795 (15.412, -42.1496) -> (16.022, -42.1496) centre (15.717, -42.1496) ccw
  arc A1796 (54.4499, -42.031) -> (55.0599, -42.031) centre (54.7549, -42.031) ccw
  arc A1797 (55.0599, -42.031) -> (54.4499, -42.031) centre (54.7549, -42.031) ccw
  arc A1798 (47.9018, -45.4206) -> (48.5118, -45.4206) centre (48.2068, -45.4206) ccw
  arc A1799 (48.5118, -45.4206) -> (47.9018, -45.4206) centre (48.2068, -45.4206) ccw
  arc A1800 (-184.4938, -61.9868) -> (-185.1038, -61.9868) centre (-184.7988, -61.9868) ccw
  arc A1801 (-185.1038, -61.9868) -> (-184.4938, -61.9868) centre (-184.7988, -61.9868) ccw
  arc A1802 (67.5639, -60.1981) -> (68.1739, -60.1981) centre (67.8689, -60.1981) ccw
  arc A1803 (68.1739, -60.1981) -> (67.5639, -60.1981) centre (67.8689, -60.1981) ccw
  arc A1804 (74.2801, -61.257) -> (73.6701, -61.257) centre (73.9751, -61.257) ccw
  arc A1805 (73.6701, -61.257) -> (74.2801, -61.257) centre (73.9751, -61.257) ccw
  arc A1806 (-190.0958, -64.7511) -> (-190.7058, -64.7511) centre (-190.4008, -64.7511) ccw
  arc A1807 (-190.7058, -64.7511) -> (-190.0958, -64.7511) centre (-190.4008, -64.7511) ccw
  arc A1808 (-159.4974, -62.8072) -> (-160.1074, -62.8072) centre (-159.8024, -62.8072) ccw
  arc A1809 (-160.1074, -62.8072) -> (-159.4974, -62.8072) centre (-159.8024, -62.8072) ccw
  arc A1810 (-163.62, -87.6421) -> (-163.01, -87.6421) centre (-163.315, -87.6421) ccw
  arc A1811 (-163.01, -87.6421) -> (-163.62, -87.6421) centre (-163.315, -87.6421) ccw
  arc A1812 (-116.8464, -62.411) -> (-117.4564, -62.411) centre (-117.1514, -62.411) ccw
  arc A1813 (-117.4564, -62.411) -> (-116.8464, -62.411) centre (-117.1514, -62.411) ccw
  arc A1814 (-99.4969, -62.411) -> (-100.1069, -62.411) centre (-99.8019, -62.411) ccw
  arc A1815 (-100.1069, -62.411) -> (-99.4969, -62.411) centre (-99.8019, -62.411) ccw
  arc A1816 (67.4526, -83.8727) -> (66.8426, -83.8727) centre (67.1476, -83.8727) ccw
  arc A1817 (66.8426, -83.8727) -> (67.4526, -83.8727) centre (67.1476, -83.8727) ccw
  arc A1818 (-54.907, -83.8839) -> (-54.297, -83.8839) centre (-54.602, -83.8839) ccw
  arc A1819 (-54.297, -83.8839) -> (-54.907, -83.8839) centre (-54.602, -83.8839) ccw
  arc A1820 (4.6329, -84.2367) -> (4.0229, -84.2367) centre (4.3279, -84.2367) ccw
  arc A1821 (4.0229, -84.2367) -> (4.6329, -84.2367) centre (4.3279, -84.2367) ccw
  arc A1822 (-60.4677, -48.7531) -> (-61.0777, -48.7531) centre (-60.7727, -48.7531) ccw
  arc A1823 (-61.0777, -48.7531) -> (-60.4677, -48.7531) centre (-60.7727, -48.7531) ccw
  arc A1824 (50.9955, -50.7221) -> (51.6055, -50.7221) centre (51.3005, -50.7221) ccw
  arc A1825 (51.6055, -50.7221) -> (50.9955, -50.7221) centre (51.3005, -50.7221) ccw
  arc A1826 (-32.3094, -57.7719) -> (-32.9194, -57.7719) centre (-32.6144, -57.7719) ccw
  arc A1827 (-32.9194, -57.7719) -> (-32.3094, -57.7719) centre (-32.6144, -57.7719) ccw
  arc A1828 (-8.0322, -57.7719) -> (-7.4222, -57.7719) centre (-7.7272, -57.7719) ccw
  arc A1829 (-7.4222, -57.7719) -> (-8.0322, -57.7719) centre (-7.7272, -57.7719) ccw
  arc A1830 (-51.177, -111.9929) -> (-50.567, -111.9929) centre (-50.872, -111.9929) ccw
  arc A1831 (-50.567, -111.9929) -> (-51.177, -111.9929) centre (-50.872, -111.9929) ccw
  arc A1832 (-144.2961, -111.9929) -> (-143.6861, -111.9929) centre (-143.9911, -111.9929) ccw
  arc A1833 (-143.6861, -111.9929) -> (-144.2961, -111.9929) centre (-143.9911, -111.9929) ccw
  arc A1834 (3.7729, -52.237) -> (3.1629, -52.237) centre (3.4679, -52.237) ccw
  arc A1835 (3.1629, -52.237) -> (3.7729, -52.237) centre (3.4679, -52.237) ccw
  arc A1836 (-145.1447, -63.5883) -> (-144.5347, -63.5883) centre (-144.8397, -63.5883) ccw
  arc A1837 (-144.5347, -63.5883) -> (-145.1447, -63.5883) centre (-144.8397, -63.5883) ccw
  arc A1838 (55.413, -86.2377) -> (54.8029, -86.2377) centre (55.108, -86.2377) ccw
  arc A1839 (54.8029, -86.2377) -> (55.413, -86.2377) centre (55.108, -86.2377) ccw
  arc A1840 (-173.981, -89.0734) -> (-174.591, -89.0734) centre (-174.286, -89.0734) ccw
  arc A1841 (-174.591, -89.0734) -> (-173.981, -89.0734) centre (-174.286, -89.0734) ccw
  arc A1842 (-148.386, -84.5438) -> (-147.776, -84.5438) centre (-148.081, -84.5438) ccw
  arc A1843 (-147.776, -84.5438) -> (-148.386, -84.5438) centre (-148.081, -84.5438) ccw
  arc A1844 (53.9321, -85.6949) -> (53.3221, -85.6949) centre (53.6271, -85.6949) ccw
  arc A1845 (53.3221, -85.6949) -> (53.9321, -85.6949) centre (53.6271, -85.6949) ccw
  arc A1846 (-116.8389, -53.2304) -> (-116.2289, -53.2304) centre (-116.5339, -53.2304) ccw
  arc A1847 (-116.2289, -53.2304) -> (-116.8389, -53.2304) centre (-116.5339, -53.2304) ccw
  arc A1848 (-54.4959, -86.4102) -> (-55.1059, -86.4102) centre (-54.8009, -86.4102) ccw
  arc A1849 (-55.1059, -86.4102) -> (-54.4959, -86.4102) centre (-54.8009, -86.4102) ccw
  arc A1850 (-53.4466, -52.8227) -> (-54.0566, -52.8227) centre (-53.7516, -52.8227) ccw
  arc A1851 (-54.0566, -52.8227) -> (-53.4466, -52.8227) centre (-53.7516, -52.8227) ccw
  arc A1852 (24.304, -52.8227) -> (23.694, -52.8227) centre (23.999, -52.8227) ccw
  arc A1853 (23.694, -52.8227) -> (24.304, -52.8227) centre (23.999, -52.8227) ccw
  arc A1854 (-52.4231, -95.9764) -> (-51.8131, -95.9764) centre (-52.1181, -95.9764) ccw
  arc A1855 (-51.8131, -95.9764) -> (-52.4231, -95.9764) centre (-52.1181, -95.9764) ccw
  arc A1856 (-39.7466, -95.9764) -> (-40.3566, -95.9764) centre (-40.0516, -95.9764) ccw
  arc A1857 (-40.3566, -95.9764) -> (-39.7466, -95.9764) centre (-40.0516, -95.9764) ccw
  arc A1858 (-52.8311, -51.2215) -> (-53.4411, -51.2215) centre (-53.1361, -51.2215) ccw
  arc A1859 (-53.4411, -51.2215) -> (-52.8311, -51.2215) centre (-53.1361, -51.2215) ccw
  arc A1860 (-20.2885, -93.1356) -> (-19.6785, -93.1356) centre (-19.9835, -93.1356) ccw
  arc A1861 (-19.6785, -93.1356) -> (-20.2885, -93.1356) centre (-19.9835, -93.1356) ccw
  arc A1862 (1.7226, -93.1356) -> (1.1126, -93.1356) centre (1.4176, -93.1356) ccw
  arc A1863 (1.1126, -93.1356) -> (1.7226, -93.1356) centre (1.4176, -93.1356) ccw
  arc A1864 (-20.3708, -116.5857) -> (-19.7608, -116.5857) centre (-20.0658, -116.5857) ccw
  arc A1865 (-19.7608, -116.5857) -> (-20.3708, -116.5857) centre (-20.0658, -116.5857) ccw
  arc A1866 (-23.4046, -114.5009) -> (-22.7946, -114.5009) centre (-23.0996, -114.5009) ccw
  arc A1867 (-22.7946, -114.5009) -> (-23.4046, -114.5009) centre (-23.0996, -114.5009) ccw
  arc A1868 (-82.163, -114.5009) -> (-81.553, -114.5009) centre (-81.858, -114.5009) ccw
  arc A1869 (-81.553, -114.5009) -> (-82.163, -114.5009) centre (-81.858, -114.5009) ccw
  arc A1870 (-12.2538, -115.6266) -> (-12.8638, -115.6266) centre (-12.5588, -115.6266) ccw
  arc A1871 (-12.8638, -115.6266) -> (-12.2538, -115.6266) centre (-12.5588, -115.6266) ccw
  arc A1872 (-23.3147, -105.8847) -> (-22.7046, -105.8847) centre (-23.0097, -105.8847) ccw
  arc A1873 (-22.7046, -105.8847) -> (-23.3147, -105.8847) centre (-23.0097, -105.8847) ccw
  arc A1874 (75.6538, -9.034) -> (76.2639, -9.034) centre (75.9589, -9.034) ccw
  arc A1875 (76.2639, -9.034) -> (75.6538, -9.034) centre (75.9589, -9.034) ccw
  arc A1876 (6.5454, -83.224) -> (7.1554, -83.224) centre (6.8504, -83.224) ccw
  arc A1877 (7.1554, -83.224) -> (6.5454, -83.224) centre (6.8504, -83.224) ccw
  arc A1878 (-132.2824, -64.4897) -> (-131.6724, -64.4897) centre (-131.9774, -64.4897) ccw
  arc A1879 (-131.6724, -64.4897) -> (-132.2824, -64.4897) centre (-131.9774, -64.4897) ccw
  line L316 (-180.518, 18.453) -> (-184.318, 18.453)
  line L317 (-184.318, 18.453) -> (-184.318, 22.253)
  line L318 (-180.518, 22.253) -> (-180.518, 18.453)
  line L319 (-184.318, 22.253) -> (-180.518, 22.253)
  arc A1880 (-180.5461, 25.047) -> (-184.5339, 25.047) centre (-182.54, 25.047) ccw
  arc A1881 (-184.5339, 25.047) -> (-180.5461, 25.047) centre (-182.54, 25.047) ccw
  arc A1882 (-176.6091, 24.92) -> (-178.3109, 24.92) centre (-177.46, 24.92) ccw
  arc A1883 (-178.3109, 24.92) -> (-176.6091, 24.92) centre (-177.46, 24.92) ccw
  arc A1884 (-188.4709, 24.92) -> (-186.7691, 24.92) centre (-187.62, 24.92) ccw
  arc A1885 (-186.7691, 24.92) -> (-188.4709, 24.92) centre (-187.62, 24.92) ccw
  line L320 (-150.518, 22.253) -> (-150.518, 18.453)
  line L321 (-154.318, 18.453) -> (-154.318, 22.253)
  line L322 (-150.518, 18.453) -> (-154.318, 18.453)
  line L323 (-154.318, 22.253) -> (-150.518, 22.253)
  arc A1886 (-154.5339, 25.047) -> (-150.5461, 25.047) centre (-152.54, 25.047) ccw
  arc A1887 (-150.5461, 25.047) -> (-154.5339, 25.047) centre (-152.54, 25.047) ccw
  arc A1888 (-148.3109, 24.92) -> (-146.6091, 24.92) centre (-147.46, 24.92) ccw
  arc A1889 (-146.6091, 24.92) -> (-148.3109, 24.92) centre (-147.46, 24.92) ccw
  arc A1890 (-156.7691, 24.92) -> (-158.4709, 24.92) centre (-157.62, 24.92) ccw
  arc A1891 (-158.4709, 24.92) -> (-156.7691, 24.92) centre (-157.62, 24.92) ccw
  line L324 (-120.518, 22.253) -> (-120.518, 18.453)
  line L325 (-120.518, 18.453) -> (-124.318, 18.453)
  line L326 (-124.318, 22.253) -> (-120.518, 22.253)
  line L327 (-124.318, 18.453) -> (-124.318, 22.253)
  arc A1892 (-124.5339, 25.047) -> (-120.5461, 25.047) centre (-122.54, 25.047) ccw
  arc A1893 (-120.5461, 25.047) -> (-124.5339, 25.047) centre (-122.54, 25.047) ccw
  arc A1894 (-118.3109, 24.92) -> (-116.6091, 24.92) centre (-117.46, 24.92) ccw
  arc A1895 (-116.6091, 24.92) -> (-118.3109, 24.92) centre (-117.46, 24.92) ccw
  arc A1896 (-126.7691, 24.92) -> (-128.4709, 24.92) centre (-127.62, 24.92) ccw
  arc A1897 (-128.4709, 24.92) -> (-126.7691, 24.92) centre (-127.62, 24.92) ccw
  line L328 (-90.518, 22.253) -> (-90.518, 18.453)
  line L329 (-94.318, 18.453) -> (-94.318, 22.253)
  line L330 (-94.318, 22.253) -> (-90.518, 22.253)
  line L331 (-90.518, 18.453) -> (-94.318, 18.453)
  arc A1898 (-90.5461, 25.047) -> (-94.5339, 25.047) centre (-92.54, 25.047) ccw
  arc A1899 (-94.5339, 25.047) -> (-90.5461, 25.047) centre (-92.54, 25.047) ccw
  arc A1900 (-86.6091, 24.92) -> (-88.3109, 24.92) centre (-87.46, 24.92) ccw
  arc A1901 (-88.3109, 24.92) -> (-86.6091, 24.92) centre (-87.46, 24.92) ccw
  arc A1902 (-96.7691, 24.92) -> (-98.4709, 24.92) centre (-97.62, 24.92) ccw
  arc A1903 (-98.4709, 24.92) -> (-96.7691, 24.92) centre (-97.62, 24.92) ccw
  line L332 (-60.518, 22.253) -> (-60.518, 18.453)
  line L333 (-60.518, 18.453) -> (-64.318, 18.453)
  line L334 (-64.318, 22.253) -> (-60.518, 22.253)
  line L335 (-64.318, 18.453) -> (-64.318, 22.253)
  arc A1904 (-60.5461, 25.047) -> (-64.5339, 25.047) centre (-62.54, 25.047) ccw
  arc A1905 (-64.5339, 25.047) -> (-60.5461, 25.047) centre (-62.54, 25.047) ccw
  arc A1906 (-58.3109, 24.92) -> (-56.6091, 24.92) centre (-57.46, 24.92) ccw
  arc A1907 (-56.6091, 24.92) -> (-58.3109, 24.92) centre (-57.46, 24.92) ccw
  arc A1908 (-68.4709, 24.92) -> (-66.7691, 24.92) centre (-67.62, 24.92) ccw
  arc A1909 (-66.7691, 24.92) -> (-68.4709, 24.92) centre (-67.62, 24.92) ccw
  line L336 (-34.318, 22.253) -> (-30.518, 22.253)
  line L337 (-34.318, 18.453) -> (-34.318, 22.253)
  line L338 (-30.518, 22.253) -> (-30.518, 18.453)
  line L339 (-30.518, 18.453) -> (-34.318, 18.453)
  arc A1910 (-34.5339, 25.047) -> (-30.5461, 25.047) centre (-32.54, 25.047) ccw
  arc A1911 (-30.5461, 25.047) -> (-34.5339, 25.047) centre (-32.54, 25.047) ccw
  arc A1912 (-26.6091, 24.92) -> (-28.3109, 24.92) centre (-27.46, 24.92) ccw
  arc A1913 (-28.3109, 24.92) -> (-26.6091, 24.92) centre (-27.46, 24.92) ccw
  arc A1914 (-38.4709, 24.92) -> (-36.7691, 24.92) centre (-37.62, 24.92) ccw
  arc A1915 (-36.7691, 24.92) -> (-38.4709, 24.92) centre (-37.62, 24.92) ccw
  line L340 (-4.318, 18.453) -> (-4.318, 22.253)
  line L341 (-0.518, 22.253) -> (-0.518, 18.453)
  line L342 (-4.318, 22.253) -> (-0.518, 22.253)
  line L343 (-0.518, 18.453) -> (-4.318, 18.453)
  arc A1916 (-4.5339, 25.047) -> (-0.5461, 25.047) centre (-2.54, 25.047) ccw
  arc A1917 (-0.5461, 25.047) -> (-4.5339, 25.047) centre (-2.54, 25.047) ccw
  arc A1918 (3.3909, 24.92) -> (1.6891, 24.92) centre (2.54, 24.92) ccw
  arc A1919 (1.6891, 24.92) -> (3.3909, 24.92) centre (2.54, 24.92) ccw
  arc A1920 (-8.4709, 24.92) -> (-6.7691, 24.92) centre (-7.62, 24.92) ccw
  arc A1921 (-6.7691, 24.92) -> (-8.4709, 24.92) centre (-7.62, 24.92) ccw
  line L344 (25.682, 18.453) -> (25.682, 22.253)
  line L345 (25.682, 22.253) -> (29.482, 22.253)
  line L346 (29.482, 22.253) -> (29.482, 18.453)
  line L347 (29.482, 18.453) -> (25.682, 18.453)
  arc A1922 (25.4661, 25.047) -> (29.4539, 25.047) centre (27.46, 25.047) ccw
  arc A1923 (29.4539, 25.047) -> (25.4661, 25.047) centre (27.46, 25.047) ccw
  arc A1924 (33.3909, 24.92) -> (31.6891, 24.92) centre (32.54, 24.92) ccw
  arc A1925 (31.6891, 24.92) -> (33.3909, 24.92) centre (32.54, 24.92) ccw
  arc A1926 (21.5291, 24.92) -> (23.2309, 24.92) centre (22.38, 24.92) ccw
  arc A1927 (23.2309, 24.92) -> (21.5291, 24.92) centre (22.38, 24.92) ccw
  line L348 (-180.518, -11.547) -> (-184.318, -11.547)
  line L349 (-184.318, -11.547) -> (-184.318, -7.747)
  line L350 (-184.318, -7.747) -> (-180.518, -7.747)
  line L351 (-180.518, -7.747) -> (-180.518, -11.547)
  arc A1928 (-180.5461, -4.953) -> (-184.5339, -4.953) centre (-182.54, -4.953) ccw
  arc A1929 (-184.5339, -4.953) -> (-180.5461, -4.953) centre (-182.54, -4.953) ccw
  arc A1930 (-176.6091, -5.08) -> (-178.3109, -5.08) centre (-177.46, -5.08) ccw
  arc A1931 (-178.3109, -5.08) -> (-176.6091, -5.08) centre (-177.46, -5.08) ccw
  arc A1932 (-186.7691, -5.08) -> (-188.4709, -5.08) centre (-187.62, -5.08) ccw
  arc A1933 (-188.4709, -5.08) -> (-186.7691, -5.08) centre (-187.62, -5.08) ccw
  line L352 (-154.318, -11.547) -> (-154.318, -7.747)
  line L353 (-150.518, -7.747) -> (-150.518, -11.547)
  line L354 (-154.318, -7.747) -> (-150.518, -7.747)
  line L355 (-150.518, -11.547) -> (-154.318, -11.547)
  arc A1934 (-150.5461, -4.953) -> (-154.5339, -4.953) centre (-152.54, -4.953) ccw
  arc A1935 (-154.5339, -4.953) -> (-150.5461, -4.953) centre (-152.54, -4.953) ccw
  arc A1936 (-148.3109, -5.08) -> (-146.6091, -5.08) centre (-147.46, -5.08) ccw
  arc A1937 (-146.6091, -5.08) -> (-148.3109, -5.08) centre (-147.46, -5.08) ccw
  arc A1938 (-158.4709, -5.08) -> (-156.7691, -5.08) centre (-157.62, -5.08) ccw
  arc A1939 (-156.7691, -5.08) -> (-158.4709, -5.08) centre (-157.62, -5.08) ccw
  line L356 (-120.518, -7.747) -> (-120.518, -11.547)
  line L357 (-120.518, -11.547) -> (-124.318, -11.547)
  line L358 (-124.318, -7.747) -> (-120.518, -7.747)
  line L359 (-124.318, -11.547) -> (-124.318, -7.747)
  arc A1940 (-124.5339, -4.953) -> (-120.5461, -4.953) centre (-122.54, -4.953) ccw
  arc A1941 (-120.5461, -4.953) -> (-124.5339, -4.953) centre (-122.54, -4.953) ccw
  arc A1942 (-116.6091, -5.08) -> (-118.3109, -5.08) centre (-117.46, -5.08) ccw
  arc A1943 (-118.3109, -5.08) -> (-116.6091, -5.08) centre (-117.46, -5.08) ccw
  arc A1944 (-126.7691, -5.08) -> (-128.4709, -5.08) centre (-127.62, -5.08) ccw
  arc A1945 (-128.4709, -5.08) -> (-126.7691, -5.08) centre (-127.62, -5.08) ccw